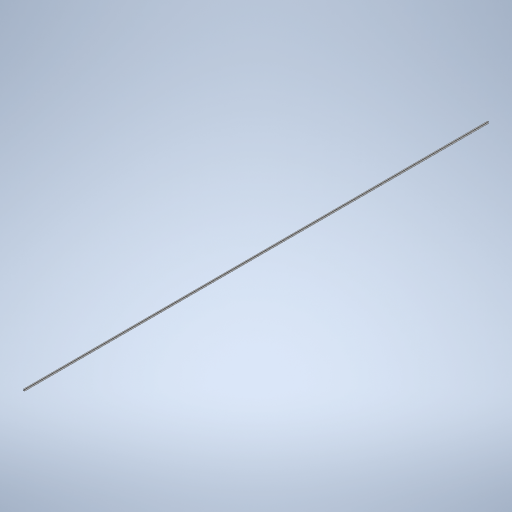
# Autodesk Inventor part: Rail48in
Saved by Autodesk Inventor 2023 (Build 270158030, 158C)
## iProperties
Created: 2023-02-14
Part Number: Rail48in
Material: Generic
Document SubType Name: Modeling
Designer: jeremyy
Density: 1 g/cm^3
Appearance: Default
Author: jeremyy
Autodesk Inventor part; units mm, degrees
ref_plane "YZ Plane" through (0, 0, 0) normal (1, 0, 0) x (0, 1, 0)
ref_plane "XZ Plane" through (0, 0, 0) normal (0, 1, 0) x (-1, 0, 0)
ref_plane "XY Plane" through (0, 0, 0) normal (0, 0, 1) x (1, 0, 0)
sketch "Sketch1" plane through (0, 0, 0) normal (0, 0, 1) x (1, 0, 0)
  line L0 (0, 0) -> (3.7042, 0)
  line L1 (1.8521, 0) -> (1.8521, 0.6615)
  line L2 (1.8521, 0.6615) -> (2.1167, 0.6615)
  line L3 (2.1167, 0.6615) -> (3.7042, 0.295)
  line L4 (3.7042, 0.295) -> (3.7042, 0)
  line L5 (1.8521, 0.6615) -> (1.8521, 2.7781)
  line L6 (1.8521, 2.7781) -> (2.1167, 2.7781)
  line L7 (2.1167, 2.7781) -> (2.1167, 0.6615)
  line L8 (1.8521, 2.7781) -> (1.8521, 3.8365)
  line L9 (1.8521, 3.8365) -> (2.8549, 3.8365)
  line L10 (2.1167, 2.7781) -> (3.1089, 3.0072)
  line L11 (2.1167, 2.7781) -> (3.135, 2.7781) construction
  line L12 (3.1089, 3.5825) -> (3.1089, 3.0072)
  arc A0 (3.1089, 3.5825) -> (2.8549, 3.8365) centre (2.8549, 3.5825) ccw
  line L13 (3.7042, 0) -> (0, 0)
  line L14 (1.8521, 0.6615) -> (1.5875, 0.6615)
  line L15 (1.5875, 0.6615) -> (0, 0.295)
  line L16 (0, 0.295) -> (0, 0)
  line L17 (1.8521, 2.7781) -> (1.5875, 2.7781)
  line L18 (1.5875, 2.7781) -> (1.5875, 0.6615)
  line L19 (1.8521, 3.8365) -> (0.8493, 3.8365)
  line L20 (1.5875, 2.7781) -> (0.5953, 3.0072)
  line L21 (1.5875, 2.7781) -> (0.5692, 2.7781) construction
  line L22 (0.5953, 3.5825) -> (0.5953, 3.0072)
  arc A1 (0.8493, 3.8365) -> (0.5953, 3.5825) centre (0.8493, 3.5825) ccw
  dimension "d3" = 0.6615
  dimension "d4" = 0.2646
  dimension "d5" = 167
  dimension "d6" = 2.1167
  dimension "d7" = 1.0583
  dimension "d9" = 13
  dimension "d10" = 0.254
  constraints: 46 end point, 10 symmetric about line, 4 perpendicular, 4 point on circle, 3 vertical, 2 centre point, 2 horizontal, 2 parallel, 2 tangent, 1 equal length, 1 midpoint, 1 other
  measures "d3" distance of L1.start L1.end
  measures "d4" distance of L1.end L2.end
  measures "d5" angle of L2 L3
  measures "d6" distance of L1.end L5.end
  measures "d7" distance of L5.end L8.end
  measures "d9" angle of L11 L10
  measures "d10" radius of A0
extrude "Extrusion1" add sketch "Sketch1" against normal blind 1219.2
body "Solid1"
